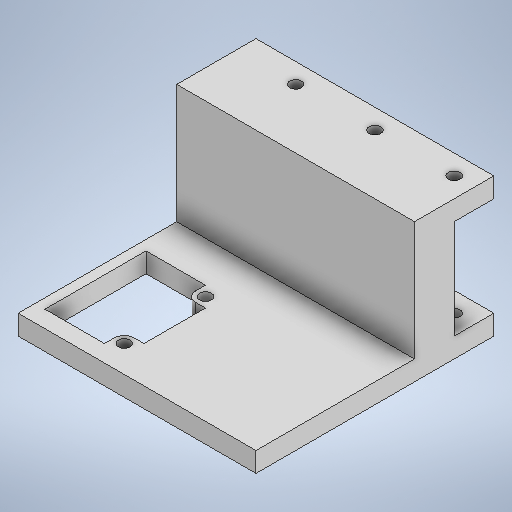
# Autodesk Inventor part: Battery_zig
Saved by Autodesk Inventor 2025 (Build 290162010, 162A)
## iProperties
Created: 2024-09-12
Part Number: Battery_zig
Material: Generic
Document SubType Name: Modeling
Designer: fist5
Density: 1 g/cm^3
Appearance: Default
Author: fist5
Autodesk Inventor part; units mm, degrees
ref_plane "YZ Plane" through (0, 0, 0) normal (1, 0, 0) x (0, 1, 0)
ref_plane "XZ Plane" through (0, 0, 0) normal (0, 1, 0) x (-1, 0, 0)
ref_plane "XY Plane" through (0, 0, 0) normal (0, 0, 1) x (1, 0, 0)
sketch "Sketch1" plane through (0, 0, 0) normal (0, 1, 0) x (-1, 0, 0)
  line L0 (45, -43) -> (-45, -43)
  line L1 (-45, -43) -> (-45, 43)
  line L2 (-45, 43) -> (45, 43)
  line L3 (45, 43) -> (45, -43)
  line L4 (45, -43) -> (-45, 43) construction
  line L5 (-45, -43) -> (45, 43) construction
  line L6 (-45, -43) -> (15, -43)
  line L7 (15, -43) -> (15, 17)
  line L8 (15, 17) -> (-45, 17)
  line L9 (-45, 17) -> (-45, -43)
  point P0 (0, 0)
  point P1 (-45, -13)
  point P2 (-45, 17)
  dimension "d0" = 90
  dimension "d1" = 86
  dimension "d68" = 60
  dimension "d69" = 60
  constraints: 20 end point, 4 parallel, 3 midpoint, 2 horizontal, 2 perpendicular
  measures "d0" distance between parallel lines of L1 L3
  measures "d1" distance between parallel lines of L2 L0
  measures "d68" distance from line of point (-45, -13) L7
  measures "d69" distance between parallel lines of L0 L8
extrude "Extrusion1" add sketch "Sketch1" along normal blind 5 contours L0 L1 L8 L7
sketch "Sketch2" plane through (0, 5, 0) normal (0, 1, 0) x (1, 0, 0)
  line L0 (-45, 43) -> (-45, -43) projected
  line L1 (45, -17) -> (45, 43) projected
  line L2 (-15, 33) -> (45, 33)
  line L3 (45, 33) -> (45, 23)
  line L4 (45, 23) -> (-15, 23)
  line L5 (45, -23) -> (45, -33)
  line L6 (-45, -33) -> (-45, -23)
  line L7 (45, -17) -> (45, 43) projected
  line L8 (-15, -17) -> (45, -17) projected
  line L9 (-15, 43) -> (-15, -17) projected
  line L10 (45, 43) -> (-15, 43) projected
  point P0 (0, 0)
  point P1 (45, -43)
  point P2 (45, 0)
  point P3 (-45, 23)
  point P4 (45, 33)
  point P5 (-15, 33)
  point P6 (-15, 23)
  dimension "d5" = 23
  dimension "d6" = 10
  constraints: 10 end point, 5 point on line, 2 parallel, 1 horizontal, 1 horizontal alignment, 1 perpendicular
  measures "d5" distance of L3.end point (45, 0)
  measures "d6" distance between parallel lines of L4 L2
extrude "Extrusion2" add sketch "Sketch2" along normal blind 30 contours L4 L9 L2 L1
sketch "Sketch3" plane through (45, 5, -33) normal (0, 0, -1) x (-1, 0, 0)
  line L0 (0, 0) -> (0, 30) projected
  line L1 (90, 0) -> (90, 30) projected
  line L2 (0, 30) -> (60, 30)
  line L3 (60, 25) -> (0, 25)
  line L4 (0, 25) -> (0, 30)
  line L5 (0, 0) -> (60, 0) projected
  line L6 (0, 0) -> (0, 30) projected
  line L7 (60, 30) -> (0, 30) projected
  line L8 (60, 0) -> (60, 30) projected
  point P0 (45, -5)
  point P1 (0, 25)
  dimension "d10" = 5
  constraints: 6 end point, 2 point on line, 1 horizontal, 1 parallel
  measures "d10" distance between parallel lines of L2 L3
extrude "Extrusion3" add sketch "Sketch3" along normal blind 10 contours L0 L2 L8 L3
sketch "Sketch5" plane through (0, 35, 0) normal (0, 1, 0) x (1, 0, 0)
  circle A0 centre (40, 38) radius 1.5
  line L0 (-15, 43) -> (45, 43) projected
  line L1 (45, 23) -> (45, 43) projected
  circle A1 centre (20, 38) radius 1.5
  circle A2 centre (0, 38) radius 1.5
  point P0 (0, 0)
  point P1 (-45, 43)
  dimension "d15" = 3
  dimension "d21" = 5
  dimension "d22" = 5
  dimension "d28" = 20
  constraints: 3 centre point, 1 horizontal, 1 vertical, 4 other
  measures "d15" diameter of A0
  measures "d21" distance from line of L0 A0.centre
  measures "d22" distance from line of L1 A0.centre
  measures "d28" distance of A0.centre A1.centre
extrude "Extrusion5" cut sketch "Sketch5" against normal up to surface (35 mm away)
sketch "Sketch8" plane through (0, 0, 0) normal (0, -1, 0) x (1, 0, 0)
  line L0 (-5, -10.25) -> (5, -10.25)
  line L1 (5, -10.25) -> (5, 10.25)
  line L2 (5, 10.25) -> (-5, 10.25)
  line L3 (-5, 10.25) -> (-5, -10.25)
  line L4 (-5, -10.25) -> (5, 10.25) construction
  line L5 (5, -10.25) -> (-5, 10.25) construction
  circle A0 centre (5, -10.25) radius 2.5
  circle A1 centre (5, 10.25) radius 2.5
  circle A2 centre (5, -10.25) radius 1.5
  circle A3 centre (5, 10.25) radius 1.5
  line L6 (7.5, 12.75) -> (-12.5, 12.75)
  line L7 (-12.5, 12.75) -> (-12.5, -12.75)
  line L8 (-12.5, -12.75) -> (7.5, -12.75)
  line L9 (7.5, -12.75) -> (7.5, 12.75)
  line L10 (2.5, -12.75) -> (2.5, 12.75)
  line L11 (7.5, -7.75) -> (-12.5, -7.75)
  line L12 (7.5, 7.75) -> (-12.5, 7.75)
  point P0 (0, 0)
  point P1 (0, 0)
  point P2 (2.5, 10.25)
  point P3 (2.5, -10.25)
  point P4 (5, -7.75)
  point P5 (5, 7.75)
  dimension "d66" = 20.5
  dimension "d67" = 10
  dimension "d70" = 5
  dimension "d71" = 5
  dimension "d74" = 3
  dimension "d75" = 3
  dimension "d76" = 20
  constraints: 26 end point, 6 coincident, 6 point on line, 6 tangent, 5 perpendicular, 4 centre point, 4 parallel, 2 horizontal, 2 midpoint
  measures "d66" distance of L1.end L0.end
  measures "d67" distance between parallel lines of L1 L3
  measures "d70" diameter of A0
  measures "d71" diameter of A1
  measures "d74" diameter of A2
  measures "d75" diameter of A3
  measures "d76" distance between parallel lines of L9 L7
extrude "Extrusion8" cut sketch "Sketch8" against normal up to surface (5 mm away) contours L3 L11 L10 L0 | L0 L10 L8 L7 L11 L3 | L10 L11 A0 | L11 L7 L12 L3 | L3 L12 L10 L11 | A2 L1 L0 | L0 L1 A2 | L11 L10 L12 L1 | L1 L12 L9 L11 | L12 L7 L6 L10 L2 L3 | L3 L2 L10 L12 | L12 L10 A1 | A3 L2 L1 | L1 L2 A3
body "Solid1"
